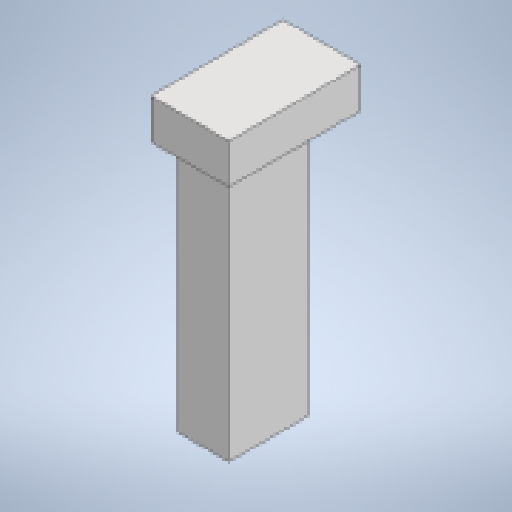
# Autodesk Inventor part: палка
Saved by Autodesk Inventor 2023 (Build 270158000, 158)
## iProperties
Created: 2025-01-24
Part Number: палка
Material: Типовые
Document SubType Name: Modeling
Designer: DELL
Density: 1 g/cm^3
Appearance: По умолчанию
Author: DELL
Autodesk Inventor part; units mm, degrees
ref_plane "YZ Plane" through (0, 0, 0) normal (1, 0, 0) x (0, 1, 0)
ref_plane "XZ Plane" through (0, 0, 0) normal (0, 1, 0) x (-1, 0, 0)
ref_plane "XY Plane" through (0, 0, 0) normal (0, 0, 1) x (1, 0, 0)
sketch "Эскиз1" plane through (0, 0, 0) normal (0, 1, 0) x (-1, 0, 0)
  line L0 (2.774, 2.3279) -> (-1.126, 2.3279)
  line L1 (-1.126, 2.3279) -> (-1.126, -3.6721)
  line L2 (-1.126, -3.6721) -> (2.774, -3.6721)
  line L3 (2.774, -3.6721) -> (2.774, 2.3279)
  point P0 (0, 0)
  dimension "d0" = 3.9
  dimension "d1" = 6
  constraints: 8 end point, 2 parallel, 1 horizontal, 1 perpendicular
  measures "d0" distance of L2.end L1.end
  measures "d1" distance of L1.end L0.end
extrude "Выдавливание1" add sketch "Эскиз1" along normal blind 20
sketch "Эскиз2" plane through (0, 20, 0) normal (0, 1, 0) x (1, 0, 0)
  line L0 (1.126, -2.3279) -> (1.126, 3.6721) projected
  line L1 (1.126, 3.6721) -> (-2.774, 3.6721) projected
  line L2 (-2.774, 3.6721) -> (-2.774, -2.3279) projected
  line L3 (-2.774, -2.3279) -> (1.126, -2.3279) projected
  line L4 (-2.774, 3.6721) -> (-2.774, 5.6721)
  line L5 (-2.774, 5.6721) -> (3.126, 5.6721)
  line L6 (3.126, 5.6721) -> (3.126, -4.3279)
  line L7 (3.126, -4.3279) -> (-2.774, -4.3279)
  line L8 (-2.774, -4.3279) -> (-2.774, -2.3279)
  dimension "d7" = 2
  dimension "d8" = 2
  dimension "d9" = 2
  constraints: 10 end point, 4 perpendicular, 1 point on line, 1 vertical
  measures "d7" distance between parallel lines of L7 L3
  measures "d8" distance between parallel lines of L6 L0
  measures "d9" distance between parallel lines of L1 L5
extrude "Выдавливание2" add sketch "Эскиз2" along normal blind 3
